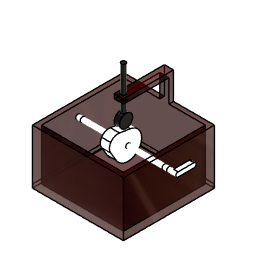
cam_follower (Autodesk Fusion 360 design; units mm, degrees)
Autodesk Fusion 360 part; units mm, degrees
sketch "Sketch1" plane through (0, 0, 0) normal (0, 0, 1) x (1, 0, 0)
  line L0 (-50, 50) -> (50, 50)
  line L1 (50, 50) -> (50, -50)
  line L2 (50, -50) -> (-50, -50)
  line L3 (-50, -50) -> (-50, 50)
  line L4 (-45, 45) -> (45, 45)
  line L5 (45, 45) -> (45, -45)
  line L6 (45, -45) -> (-45, -45)
  line L7 (-45, -45) -> (-45, 45)
  dimension "d32" = 5
  constraint horizontal L0
  constraint vertical L1
  constraint horizontal L2
  constraint vertical L3
  constraint horizontal L4
  constraint vertical L5
  constraint horizontal L6
  constraint vertical L7
  measures "d32" distance of L1 L5
extrude "Extrude1" add sketch "Sketch1" along normal blind 60 makes body 1
sketch "Sketch2" plane through (0, 0, 0) normal (0, 0, 1) x (1, 0, 0)
  line L0 (-50.0074, 50.0074) -> (49.4436, 50.0074)
  line L1 (49.4436, 50.0074) -> (49.4436, -49.4436)
  line L2 (49.4436, -49.4436) -> (-50.0074, -49.4436)
  line L3 (-50.0074, -49.4436) -> (-50.0074, 50.0074)
  constraint horizontal L0
  constraint vertical L1
  constraint horizontal L2
  constraint vertical L3
extrude "Extrude2" add sketch "Sketch2" along normal blind 4 bodies 1
sketch "Sketch3" plane through (50, 0, 0) normal (1, 0, 0) x (0, 1, 0)
  line L0 (-50, 0) -> (50, 0)
  line L1 (50, 0) -> (50, 60)
  line L2 (50, 60) -> (-50, 60)
  line L3 (-50, 60) -> (-50, 0)
  circle A0 centre (0, 43) radius 2.5
  dimension "d5" = 5
  dimension "d13" = 50
  measures "d5" diameter of A0
  measures "d13" distance of L1 A0.centre
extrude "Extrude3" cut sketch "Sketch3" against normal blind 108 contours A0 bodies 1
sketch "Sketch4" plane through (0, 0, 60) normal (0, 0, 1) x (-1, 0, 0)
  line L0 (-45, 45) -> (45, 45)
  line L1 (45, 45) -> (45, -45)
  line L2 (45, -45) -> (-45, -45)
  line L3 (-45, -45) -> (-45, 45)
  line L4 (50, 50) -> (-50, 50)
  line L5 (-50, 50) -> (-50, -50)
  line L6 (-50, -50) -> (50, -50)
  line L7 (50, -50) -> (50, 50)
  line L8 (5, -50) -> (-5, -50)
  line L9 (-5, -50) -> (-5, -45)
  line L10 (-5, -45) -> (5, -45)
  line L11 (5, -45) -> (5, -50)
  constraint horizontal L8
  constraint vertical L9
  constraint horizontal L10
  constraint vertical L11
  constraint coincident L2 L9.end
  constraint coincident L6 L8.start
extrude "Extrude4" add sketch "Sketch4" along normal blind 30 contours L2 L6 L8 L9 L10 L11 bodies 1
sketch "Sketch5" plane through (0, 45, 0) normal (0, -1, 0) x (1, 0, 0)
  line L0 (45, 4) -> (45, 60)
  line L1 (45, 60) -> (5, 60)
  line L2 (5, 60) -> (5, 90)
  line L3 (5, 90) -> (-5, 90)
  line L4 (-5, 90) -> (-5, 60)
  line L5 (-5, 60) -> (-45, 60)
  line L6 (-45, 60) -> (-45, 4)
  line L7 (-5, 90) -> (5, 90)
  line L8 (5, 90) -> (5, 85)
  line L9 (5, 85) -> (-5, 85)
  line L10 (-5, 85) -> (-5, 90)
  line L11 (-45, 4) -> (45, 4)
  constraint horizontal L7
  constraint vertical L8
  constraint horizontal L9
  constraint vertical L10
  constraint coincident L2 L8.end
  constraint coincident L3.end L4.start
extrude "Extrude5" add sketch "Sketch5" along normal blind 50 contours L2 L3 L4 L7 L8 L9 L10 bodies 1
sketch "Sketch6" plane through (0, 0, 90) normal (0, 0, 1) x (-1, 0, 0)
  line L0 (-5, 5) -> (-5, -50)
  line L1 (-5, -50) -> (5, -50)
  line L2 (5, -50) -> (5, 5)
  line L3 (5, 5) -> (-5, 5)
  line L4 (45, -45) -> (5, -45)
  line L5 (-5, -45) -> (5, -45)
  circle A0 centre (0, 0) radius 2.5
  dimension "d17" = 5
  dimension "d18" = 50
  measures "d17" diameter of A0
  measures "d18" distance of L1 A0.centre
extrude "Extrude6" cut sketch "Sketch6" against normal blind 5 contours A0 bodies 1
copy_body "Body->Comp1" bodies 1 removing the originals makes body 2 in component "Base"
sketch "Sketch1 (2)" plane through (0, 0, 4) normal (0, 0, 1) x (-1, 0, 0) in component "Base"
  line L0 (-45, 45) -> (-45, -45)
  line L1 (-45, -45) -> (45, -45)
  line L2 (45, -45) -> (45, 45)
  line L3 (45, 45) -> (-45, 45)
  line L4 (5, 45) -> (5, -45)
  line L5 (-5, 45) -> (-5, -45)
  line L6 (-5, 5) -> (5, 5)
  dimension "d22" = 40
  dimension "d23" = 40
  dimension "d24" = 10
  constraint coincident L3 L4.start
  constraint coincident L1 L4.end
  constraint perpendicular L1 L4
  constraint coincident L3 L5.start
  constraint coincident L1 L5.end
  constraint perpendicular L1 L5
  measures "d22" distance of L2 L4
  measures "d23" distance of L0 L5
  measures "d24" distance of L6.start L6.end
sketch "Sketch2 (2)" plane through (50, 0, 0) normal (1, 0, 0) x (0, 1, 0) in component "Base"
  circle A0 centre (0, 43) radius 2.5
  line L0 (-50, 0) -> (50, 0)
  line L1 (50, 0) -> (50, 60)
  line L2 (50, 60) -> (-50, 60)
  line L3 (-50, 60) -> (-50, 0)
  circle A1 centre (0, 43) radius 2.5
  constraint concentric A0 A1
extrude "Extrude1'" add sketch "Sketch2 (2)" along normal blind -40 and the other way blind -5 separate body contours A0 A1 makes body 3 in component "cam axis"
sketch "Sketch7" plane through (10, 0, 0) normal (-1, 0, 0) x (0, -1, 0)
  circle A0 centre (0, 43) radius 2.5
  circle A1 centre (0, 43) radius 15
  line L0 (-13.8306, 48.8064) -> (-9.1844, 59.8734)
  line L1 (7.8937, 60.5184) -> (13.3575, 49.8248)
  line L2 (-0.425, 65.696) -> (-0.566, 65.696)
  arc A2 (-0.425, 65.696) -> (-9.1844, 59.8734) centre (-0.425, 56.196) ccw
  arc A3 (7.8937, 60.5184) -> (-0.566, 65.696) centre (-0.566, 56.196) ccw
  dimension "d27" = 9.5
  constraint concentric A0 A1
  constraint coincident A1 L0.start
  constraint coincident A1 L1.end
  constraint tangent A1 L0
  constraint tangent A1 L1
  constraint horizontal L2
  constraint tangent L0 A2
  constraint tangent L2 A2
  constraint tangent L2 A3
  constraint tangent L1 A3
  constraint equal A2 A3
  measures "d27" radius of A2
extrude "Extrude7" add sketch "Sketch7" along normal blind 10 from surface at 5 separate body makes body 4
extrude "Extrude2'" add 1 faces at (10, 0.7601, 42.5142) along direction (-1, 0, 0) blind 40 on bodies 3 bodies 3 in component "cam axis"
extrude "Extrude3'" add 1 faces at (-30, 0.7601, 42.5142) along direction (-1, 0, 0) blind 20 on bodies 3 bodies 3 in component "cam axis"
copy_body "Body->Comp2" bodies 4 removing the originals makes body 5 in component "cam"
sketch "Sketch8" plane through (0, 0, 90) normal (0, 0, 1) x (-1, 0, 0)
  circle A0 centre (0, 0) radius 2.5
  line L0 (-5, 5) -> (-5, -50)
  line L1 (-5, -50) -> (5, -50)
  line L2 (5, -50) -> (5, 5)
  line L3 (5, 5) -> (-5, 5)
  circle A1 centre (0, 0) radius 2.5
  constraint coincident A0.centre A1.centre
sketch "Sketch9" plane through (0, 0, 90) normal (0, 0, 1) x (-1, 0, 0)
  circle A0 centre (0, 0) radius 2.5
  line L0 (-5, 5) -> (-5, -50)
  line L1 (-5, -50) -> (5, -50)
  line L2 (5, -50) -> (5, 5)
  line L3 (5, 5) -> (-5, 5)
  circle A1 centre (0, 0) radius 2.5
  constraint coincident A0.centre A1.centre
extrude "Extrude1''" add sketch "Sketch9" along normal blind 35 and the other way blind 25 separate body contours A0 A1 makes body 6 in component "follower"
sketch "Sketch11" plane through (55, 0, 0) normal (1, 0, 0) x (0, 1, 0)
  circle A0 centre (0, 43) radius 2.5
  line L0 (0, 40.4952) -> (11.5, 40.4952)
  arc A1 (11.5, 40.4952) -> (11.5, 45.4952) centre (11.5, 42.9952) ccw
  line L1 (11.5, 45.4952) -> (0, 45.4952)
  arc A2 (0, 45.4952) -> (0, 40.4952) centre (0, 42.9952) ccw
  line L2 (-2.5, 42.9952) -> (14, 42.9952) construction
  dimension "d49" = 5
  constraint tangent L0 A1
  constraint tangent A1 L1
  constraint parallel L0 L1
  constraint tangent L1 A2
  constraint tangent L0 A2
  constraint midpoint A2 L2.start
  constraint midpoint A1 L2.end
  constraint horizontal L2
  constraint coincident A0 L2.start
  measures "d49" diameter of A1
sketch "Sketch12" plane through (55, 0, 0) normal (1, 0, 0) x (0, 1, 0)
  circle A0 centre (0, 43) radius 2.5
  line L0 (-2.5, 40.5) -> (17.5, 40.5)
  arc A1 (17.5, 40.5) -> (17.5, 45.5) centre (17.5, 43) ccw
  line L1 (17.5, 45.5) -> (-2.5, 45.5)
  arc A2 (-2.5, 45.5) -> (-2.5, 40.5) centre (-2.5, 43) ccw
  line L2 (-2.5, 43) -> (17.5, 43) construction
  dimension "d56" = 5
  constraint tangent L0 A1
  constraint tangent A1 L1
  constraint parallel L0 L1
  constraint tangent L1 A2
  constraint tangent L0 A2
  constraint horizontal L2
  constraint coincident A0 A2.centre
  measures "d56" diameter of A1
extrude "Extrude6'" add sketch "Sketch12" along normal blind 5 contours A0 | A0 L0 A1 L1 bodies 3 in component "cam axis"
sketch "Sketch1 (3)" plane through (0, -2.1327, 85.9603) normal (0, 0.024803, -0.999692) x (1, 0, 0) in component "follower"
sketch "Sketch2 (3)" plane through (0, 0, 65) normal (0, 0, -1) x (1, 0, 0) in component "follower"
  circle A0 centre (0, 0) radius 2.5
  line L0 (2.508, -0.2003) -> (2.5081, 0.2997)
  line L1 (0, 0) -> (-0.2492, 0)
  line L2 (-0.2492, 0) -> (-2.5, 0)
  line L3 (2.508, -0.0003) -> (2.2829, -0.0003)
  line L4 (2.2829, -0.0003) -> (0, 0)
  line L5 (2.508, -0.0003) -> (2.5081, 0.4997)
  line L6 (2.5081, 0.2997) -> (0.0081, 0.3)
  line L7 (0.0081, 0.3) -> (0.008, -0.2)
  line L8 (0.008, -0.2) -> (2.508, -0.2003)
  line L9 (2.5081, 0.2997) -> (2.508, -0.2003)
  line L10 (0.008, -0.2) -> (-2.492, -0.1997)
  line L11 (0.0081, 0.3) -> (-2.4819, 0.3003)
  line L12 (-2.492, -0.1997) -> (-2.4819, 0.3003)
  constraint coincident A0 L2.end
  constraint coincident A0.centre L1.start
  constraint horizontal L1
  constraint perpendicular L0 L3
  constraint coincident L0 L5.end
  constraint perpendicular L3 L5
  constraint coincident L5 L0.end
  constraint perpendicular L5 L6
  constraint perpendicular L4 L7
  constraint perpendicular L0 L8
  constraint coincident L0 L3.start
  constraint coincident A0 L10.end
  constraint perpendicular L7 L10
  constraint coincident A0 L11.end
  constraint perpendicular L7 L11
extrude "Extrude3''" add sketch "Sketch2 (3)" along normal blind 1 contours L1 L2 L4 L7 L11 L12 | A0 L3 L4 L6 L7 | L1 L2 L4 L7 L10 L12 | A0 L3 L4 L7 L8 bodies 6 in component "follower"
sketch "Sketch1 (4)" plane through (0, 0, 0) normal (1, 0, 0) x (0, -0.999692, -0.024803) in component "cam axis"
sketch "Sketch3 (2)" plane through (0, 0, 0) normal (1, 0, 0) x (0, 1, 0) in component "follower"
  circle A0 centre (0, 71) radius 7.2111
extrude "Extrude4'" add sketch "Sketch3 (2)" against normal blind 3 bodies 6 in component "follower"
extrude "Extrude5'" add 1 faces at (-3, -1.6783, 66.7237) along direction (1, 0, 0) blind 5 from surface at 0.9 on bodies 6 bodies 6 in component "follower"
sketch "Sketch13" plane through (0, 1.0662, 0.0265) normal (0, -0.999692, -0.024803) x (1, 0, 0)
component "follower" placed x (1, 0, 0) y (0, 1, 0) z (0, 0, 1) at (0, 0, -5.5)
component "cam axis" placed x (1, 0, 0) y (0, 1, 0) z (0, 0, 1) at (0, 0, 0)
component "Base" placed x (1, 0, 0) y (0, 1, 0) z (0, 0, 1) at (0, 0, 0)
component "cam" placed x (1, 0, 0) y (0, -0.999692, -0.024803) z (0, 0.024803, -0.999692) at (0, -1.0665, 85.9868)
